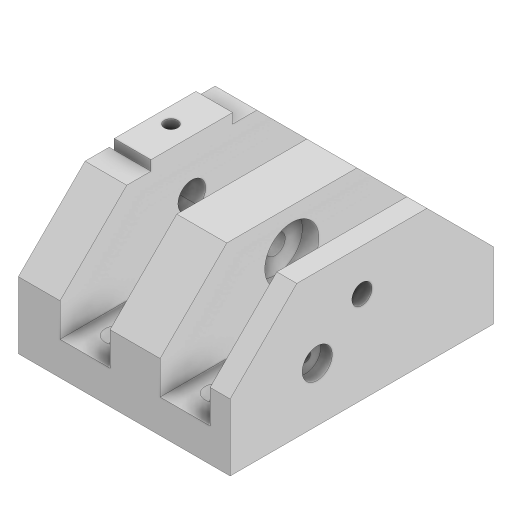
# Autodesk Inventor part: Gimbal_2
Saved by Autodesk Inventor 2023 (Build 270158000, 158)
## iProperties
Created: 2023-10-18
Part Number: Gimbal_2
Material: Generic
Document SubType Name: Modeling
Designer: MVeszpremi
Density: 1 g/cm^3
Appearance: Default
Author: MVeszpremi
Autodesk Inventor part; units mm, degrees
ref_plane "YZ Plane" through (0, 0, 0) normal (1, 0, 0) x (0, 1, 0)
ref_plane "XZ Plane" through (0, 0, 0) normal (0, 1, 0) x (-1, 0, 0)
ref_plane "XY Plane" through (0, 0, 0) normal (0, 0, 1) x (1, 0, 0)
sketch "Sketch1" plane through (0, 0, 0) normal (0, 1, 0) x (-1, 0, 0)
  line L0 (15, 30) -> (-15, 30)
  line L1 (-15, 30) -> (-15, -30)
  line L2 (-15, -30) -> (15, -30)
  line L3 (15, -30) -> (15, 30)
  line L4 (15, 30) -> (-15, -30) construction
  line L5 (-15, 30) -> (15, -30) construction
  circle A0 centre (15, 30) radius 1.5
  circle A1 centre (15, 0) radius 1.5
  circle A2 centre (15, -30) radius 1.5
  circle A3 centre (-15, -30) radius 1.5
  circle A4 centre (-15, 0) radius 1.5
  circle A5 centre (-15, 30) radius 1.5
  line L6 (22.5, 39.5) -> (-22.5, 39.5)
  line L7 (-22.5, 39.5) -> (-22.5, -39.5)
  line L8 (-22.5, -39.5) -> (22.5, -39.5)
  line L9 (22.5, -39.5) -> (22.5, 39.5)
  line L10 (22.5, 39.5) -> (-22.5, -39.5) construction
  line L11 (-22.5, 39.5) -> (22.5, -39.5) construction
  point P0 (0, 0)
  dimension "d0" = 30
  dimension "d1" = 60
  dimension "d2" = 3
  dimension "d3" = 3
  dimension "d4" = 3
  dimension "d5" = 3
  dimension "d6" = 3
  dimension "d7" = 3
  dimension "d8" = 7.5
  dimension "d9" = 9.5
  constraints: 24 end point, 6 centre point, 6 midpoint, 4 coincident, 4 parallel, 2 horizontal, 2 perpendicular
  measures "d0" distance of L0.start L0.end
  measures "d1" distance of L2.end L0.start
  measures "d2" diameter of A0
  measures "d3" diameter of A1
  measures "d4" diameter of A2
  measures "d5" diameter of A3
  measures "d6" diameter of A4
  measures "d7" diameter of A5
  measures "d8" distance between parallel lines of L3 L9
  measures "d9" distance between parallel lines of L6 L0
extrude "Extrusion1" add sketch "Sketch1" along normal blind 10 contours L0 A0 L3 A1 A2 L2 A3 L1 A4 A5 | L9 L8 L7 L6
chamfer "Chamfer1" distance 2 angle 45 6 edges at (-13.5, 10, 30) (-13.5, 10, 0) (-13.5, 10, -30) (16.5, 10, -30) (16.5, 10, 0) (16.5, 10, 30)
sketch "Sketch2" plane through (0, 0, 0) normal (0, -1, 0) x (1, 0, 0)
  line L0 (-22.5, 39.5) -> (22.5, 39.5) projected
  line L1 (22.5, 39.5) -> (28.5, 39.5)
  line L2 (28.5, 39.5) -> (28.5, -39.5)
  line L3 (28.5, -39.5) -> (22.5, -39.5)
  line L4 (22.5, -39.5) -> (22.5, 39.5)
  line L5 (-22.5, -39.5) -> (-22.5, 39.5) projected
  line L6 (-22.5, 39.5) -> (-35, 39.5)
  line L7 (-35, 39.5) -> (-35, -39.5)
  line L8 (-35, -39.5) -> (-22.5, -39.5)
  line L9 (-22.5, -39.5) -> (-22.5, 39.5)
  line L10 (22.5, -39.5) -> (-22.5, -39.5) projected
  line L11 (-7.5, 39.5) -> (7.5, 39.5)
  line L12 (7.5, 39.5) -> (7.5, -39.5)
  line L13 (7.5, -39.5) -> (-7.5, -39.5)
  line L14 (-7.5, -39.5) -> (-7.5, 39.5)
  point P0 (0, 0)
  point P1 (7.5, 39.5)
  dimension "d15" = 6
  dimension "d16" = 12.5
  dimension "d19" = 15
  dimension "d20" = 15
  constraints: 24 end point, 6 parallel, 3 horizontal, 3 perpendicular, 2 point on line
  measures "d15" distance of L0.end L1.end
  measures "d16" distance between parallel lines of L7 L5
  measures "d19" distance between parallel lines of L12 L14
  measures "d20" distance between parallel lines of L5 L14
extrude "Extrusion2" add sketch "Sketch2" against normal blind 40 contours L5 L8 L7 L6 | L0 L12 L10 L14 | L1 L2 L3 L4
sketch "Sketch3" plane through (28.5, 0, 39.5) normal (1, 0, 0) x (0, 0, -1)
  line L0 (0, 40) -> (79, 40) projected
  line L1 (39.5, 40) -> (39.5, 27.5)
  circle A0 centre (39.5, 27.5) radius 8.125
  circle A1 centre (39.5, 27.5) radius 3
  point P0 (39.5, 0)
  dimension "d21" = 16.25
  dimension "d22" = 12.5
  dimension "d23" = 6
  constraints: 2 centre point, 2 coincident, 2 end point, 1 midpoint, 1 vertical
  measures "d21" diameter of A0
  measures "d22" distance from line of L0 L1.end
  measures "d23" diameter of A1
extrude "Extrusion3" cut sketch "Sketch3" against normal blind 110.5 contours A1
chamfer "Chamfer2" distance 20 angle 45 6 edges at (25.5, 40, -39.5) (0, 40, -39.5) (-28.75, 40, -39.5) (-28.75, 40, 39.5) (0, 40, 39.5) (25.5, 40, 39.5)
sketch "Sketch4" plane through (-35, 10, -39.5) normal (-1, 0, 0) x (0, 0, 1)
  circle A0 centre (39.5, 17.5) radius 3 projected
  circle A1 centre (39.5, 17.5) radius 4.15
  line L0 (37.4354, 13.9) -> (41.5646, 13.9)
  point P0 (39.5, -10)
  dimension "d29" = 8.3
  dimension "d63" = 3.6
  constraints: 2 end point, 2 point on circle, 1 centre point, 1 coincident, 1 horizontal
  measures "d29" diameter of A1
  measures "d63" distance from line of L0 A1.centre
extrude "Extrusion4" cut sketch "Sketch4" against normal blind 15 contours A1 L0 picked at (39.6205, 14.1073)
sketch "Sketch5" plane through (-35, 10, -39.5) normal (-1, 0, 0) x (0, 0, 1)
  line L0 (35.875, 7) -> (43.125, 7)
  line L1 (43.125, 7) -> (43.125, 3.5)
  line L2 (43.125, 3.5) -> (35.875, 3.5)
  line L3 (35.875, 3.5) -> (35.875, 7)
  circle A0 centre (39.5, 17.5) radius 3 projected
  line L4 (20, 30) -> (59, 30) projected
  point P0 (39.5, -10)
  dimension "d33" = 7.25
  dimension "d34" = 3.5
  dimension "d35" = 3.625
  dimension "d36" = 23
  constraints: 8 end point, 2 parallel, 1 horizontal, 1 perpendicular
  measures "d33" distance of L0.start L0.end
  measures "d34" distance of L2.end L0.start
  measures "d35" horizontal distance of A0.centre L0.end
  measures "d36" distance from line of L4 L0.start
extrude "Extrusion5" cut sketch "Sketch5" against normal blind 15 contours L0 L1 L2 L3
sketch "Sketch6" plane through (0, 40, 0) normal (0, 1, 0) x (1, 0, 0)
  circle A0 centre (-28.75, 0) radius 2
  line L0 (-35, 19.5) -> (-35, -19.5) projected
  point P0 (0, 0)
  dimension "d42" = 4
  dimension "d43" = 6.25
  constraints: 1 centre point
  measures "d42" diameter of A0
  measures "d43" distance from line of L0 A0.centre
extrude "Extrusion6" cut sketch "Sketch6" against normal blind 15
extrude "Extrusion7" cut sketch "Sketch4" against normal blind 2 contours A0 | A1 L0 | L0 A1
sketch "Sketch7" plane through (-35, 0, -39.5) normal (-1, 0, 0) x (0, 0, 1)
  circle A0 centre (39.5, 27.5) radius 3 projected
  circle A1 centre (39.5, 27.5) radius 10.5
  circle A2 centre (39.5, 27.5) radius 17.5
  point P0 (39.5, 0)
  dimension "d46" = 21
  dimension "d47" = 35
  constraints: 2 centre point, 2 coincident
  measures "d46" diameter of A1
  measures "d47" diameter of A2
extrude "Extrusion8" cut sketch "Sketch7" against normal blind 1.5 contours A2
sketch "Sketch8" plane through (7.5, 10, 39.5) normal (1, 0, 0) x (0, 0, -1)
  circle A0 centre (39.5, 17.5) radius 3 projected
  circle A1 centre (39.5, 17.5) radius 8.125
  point P0 (39.5, -10)
  dimension "d50" = 16.25
  constraints: 1 centre point, 1 coincident
  measures "d50" diameter of A1
extrude "Extrusion9" cut sketch "Sketch8" against normal blind 5
ref_plane "Work Plane1" through (0, 10, 39.5) normal (1, 0, 0) x (0, 0, -1)
sketch "Sketch9" plane through (28.5, 0, 39.5) normal (1, 0, 0) x (0, 0, -1)
  circle A0 centre (26.0942, 16.2512) radius 4.5
  circle A1 centre (26.0942, 16.2512) radius 1.5
  circle A2 centre (39.5, 27.5) radius 3 projected
  line L0 (39.5, 27.5) -> (11.2661, 27.5)
  arc A3 (41.5646, 23.9) -> (37.4354, 23.9) centre (39.5, 27.5) ccw projected
  line L1 (39.5, 27.5) -> (26.0942, 16.2512)
  point P0 (39.5, 0)
  dimension "d53" = 9
  dimension "d54" = 3
  dimension "d55" = 17.5
  dimension "d60" = 40
  constraints: 4 end point, 2 centre point, 1 coincident, 1 horizontal
  measures "d53" diameter of A0
  measures "d54" diameter of A1
  measures "d55" distance of L0.start L1.end
  measures "d60" angle of L0 L1
extrude "Extrusion10" cut sketch "Sketch9" against normal blind 10 contours A1
extrude "Extrusion11" cut sketch "Sketch9" against normal blind 3.5 contours A0
sketch "Sketch10" plane through (0, 40, 0) normal (0, 1, 0) x (1, 0, 0)
  line L0 (-33.5, -12.2474) -> (-35, -12.2474) projected
  line L1 (-35, -12.2474) -> (-35, -19.5) projected
  line L2 (-22.5, -19.5) -> (-35, -19.5) projected
  line L3 (-22.5, -19.5) -> (-22.5, 19.5) projected
  line L4 (-35, 19.5) -> (-22.5, 19.5) projected
  line L5 (-35, 19.5) -> (-35, 12.2474) projected
  line L6 (-35, 12.2474) -> (-33.5, 12.2474) projected
  line L7 (-33.5, 12.2474) -> (-33.5, -12.2474) projected
  circle A0 centre (-28.75, 0) radius 2 projected
  line L8 (-22.5, 39.5) -> (-22.5, -39.5) projected
  line L9 (-35, 12.2474) -> (-22.5, 12.2474)
  line L10 (-22.5, 12.2474) -> (-22.5, -12.2474)
  line L11 (-22.5, -12.2474) -> (-35, -12.2474)
  line L12 (-35, -12.2474) -> (-35, 12.2474)
  point P0 (0, 0)
  constraints: 8 end point, 2 parallel, 1 horizontal, 1 perpendicular, 1 point on line
extrude "Extrusion12" add sketch "Sketch10" along normal blind 3 contours L7 L9 L3 L11
body "Solid1"
